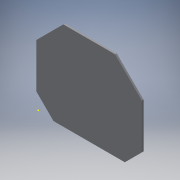
# Autodesk Inventor part: ElectronicsPlate2
Saved by Autodesk Inventor 2016 (Build 200138000, 138)
## iProperties
Created: 2016-11-05
Part Number: ElectronicsPlate2
Material: Generic
Document SubType Name: Modeling
Designer: RoboticsUser
Density: 1 g/cm^3
Appearance: Default
Mass: 159.741 g
Surface Area: 867.315 cm^2
Volume: 159.741 cm^3
Author: RoboticsUser
Autodesk Inventor part; units mm, degrees
ref_plane "YZ Plane" through (0, 0, 0) normal (1, 0, 0) x (0, 1, 0)
ref_plane "XZ Plane" through (0, 0, 0) normal (0, 1, 0) x (-1, 0, 0)
ref_plane "XY Plane" through (0, 0, 0) normal (0, 0, 1) x (1, 0, 0)
sketch "Sketch1" plane through (0, 0, 0) normal (0, 0, 1) x (1, 0, 0)
  line L0 (0, 0) -> (236.4232, 0)
  line L1 (236.4232, 0) -> (236.4232, -176.7078)
  line L2 (236.4232, -176.7078) -> (0, -176.7078)
  line L3 (0, -176.7078) -> (0, 0)
  dimension "d0" = 236.4232
  dimension "d1" = 176.7078
  constraints: 8 end point, 2 parallel, 1 horizontal, 1 perpendicular
  measures "d0" distance of L1.end L2.end
  measures "d1" distance of L0.end L1.end
extrude "Extrusion1" add sketch "Sketch1" along normal blind 3.81
chamfer "Chamfer1" distance 38.1 angle 45 1 edges at (236.4232, 0, 1.905)
chamfer "Chamfer2" distance 38.1 angle 45 1 edges at (0, 0, 1.905)
chamfer "Chamfer3" distance 38.1 angle 45 1 edges at (236.4232, -176.7078, 1.905)
chamfer "Chamfer4" distance 38.1 angle 45 1 edges at (0, -176.7078, 1.905)
move faces "Move1" translate (0, 22.098, 0) faces at (91.5077, 0, 1.27)
sketch "Sketch2" plane through (198.3232, -176.7078, 0) normal (0, -1, 0) x (1, 0, 0)
  point P0 (-198.3232, 0)
body "Solid1"
